Autodesk Inventor part; units mm, degrees
(part 2 of 2)
sketch "Sketch_86" plane through (0, 5.25, 0) normal (0, 1, 0) x (1, 0, 0)
  arc A0 (-220.5, -32) -> (-192.5, -60) centre (-192.5, -32) ccw
  line L0 (-192.5, -60) -> (192.5, -60)
  arc A1 (192.5, -60) -> (220.5, -32) centre (192.5, -32) ccw
  line L1 (220.5, -32) -> (220.5, 55)
  arc A2 (220.5, 55) -> (192.5, 83) centre (192.5, 55) ccw
  line L2 (192.5, 83) -> (-192.5, 83)
  arc A3 (-192.5, 83) -> (-220.5, 55) centre (-192.5, 55) ccw
  line L3 (-220.5, 55) -> (-220.5, -32)
  circle A4 centre (215.5, 11.5) radius 2.2
  circle A5 centre (174, -55) radius 2.2
  circle A6 centre (174, 78) radius 2.2
  circle A7 centre (60, -55) radius 2.2
  circle A8 centre (60, 78) radius 2.2
  circle A9 centre (-60, -55) radius 2.2
  circle A10 centre (-60, 78) radius 2.2
  circle A11 centre (-174, -55) radius 2.2
  circle A12 centre (-174, 78) radius 2.2
  arc A13 (-205.5, -37) -> (-197.5, -45) centre (-197.5, -37) ccw
  line L4 (-197.5, -45) -> (197.5, -45)
  arc A14 (197.5, -45) -> (205.5, -37) centre (197.5, -37) ccw
  line L5 (205.5, -37) -> (205.5, 60)
  arc A15 (205.5, 60) -> (197.5, 68) centre (197.5, 60) ccw
  line L6 (197.5, 68) -> (-197.5, 68)
  arc A16 (-197.5, 68) -> (-205.5, 60) centre (-197.5, 60) ccw
  line L7 (-205.5, 60) -> (-205.5, -37)
  circle A17 centre (-215.5, 11.5) radius 2.2
  constraints: 18 centre point, 16 end point, 16 point on circle
extrude "Extrusion31" add sketch "Sketch_86" against normal blind 1.25
sketch "Sketch_83" plane through (0, 0, 12.25) normal (0, 0, 1) x (1, 0, 0)
  line L0 (248.75, 17.25) -> (228.35, 17.25)
  line L1 (228.35, 17.25) -> (228.35, 20.483)
  line L2 (228.35, 20.483) -> (229.117, 21.25)
  line L3 (229.117, 21.25) -> (243.35, 21.25)
  line L4 (243.35, 21.25) -> (243.35, 23)
  line L5 (243.35, 23) -> (244.25, 23)
  line L6 (244.25, 23) -> (244.25, 24.25)
  line L7 (244.25, 24.25) -> (246.75, 24.25)
  line L8 (246.75, 24.25) -> (247.95, 22.25)
  line L9 (247.95, 22.25) -> (248.75, 22.25)
  line L10 (248.75, 22.25) -> (248.75, 17.25)
  line L11 (248.75, 17.25) -> (228.35, 17.25)
  constraints: 24 end point
revolve "Revolution35" add sketch "Sketch_83" angle 360 about axis through (248.75, 17.25, 12.25) along (-1, 0, 0)
thread "Thread5" size "M8x1.25" class "6g" standard "ISO Metric profile" length 12.983
sketch "Sketch_108" plane through (0, 0, 89.25) normal (0, 0, 1) x (1, 0, 0)
  line L0 (232.65, 437.5) -> (226.45, 437.5)
  line L1 (226.45, 437.5) -> (226.45, 442)
  line L2 (226.45, 442) -> (228.25, 442)
  line L3 (228.25, 442) -> (228.25, 440.5)
  line L4 (228.25, 440.5) -> (228.95, 440.5)
  line L5 (228.95, 440.5) -> (228.95, 440)
  line L6 (228.95, 440) -> (232.1595, 440)
  line L7 (232.1595, 440) -> (232.65, 439.5095)
  line L8 (232.65, 439.5095) -> (232.65, 437.5)
  line L9 (232.65, 437.5) -> (226.45, 437.5)
  constraints: 20 end point
revolve "Revolution36" add sketch "Sketch_108" angle 360 about axis through (232.65, 437.5, 89.25) along (1, 0, 0)
thread "Thread6" size "M5x0.8" class "6g" standard "ISO Metric profile" full length
sketch "Sketch_109" plane through (0, 0, 89.25) normal (0, 0, 1) x (1, 0, 0)
  line L0 (232.65, 62.5) -> (226.45, 62.5)
  line L1 (226.45, 62.5) -> (226.45, 67)
  line L2 (226.45, 67) -> (228.25, 67)
  line L3 (228.25, 67) -> (228.25, 65.5)
  line L4 (228.25, 65.5) -> (228.95, 65.5)
  line L5 (228.95, 65.5) -> (228.95, 65)
  line L6 (228.95, 65) -> (232.1595, 65)
  line L7 (232.1595, 65) -> (232.65, 64.5095)
  line L8 (232.65, 64.5095) -> (232.65, 62.5)
  line L9 (232.65, 62.5) -> (226.45, 62.5)
  constraints: 20 end point
revolve "Revolution37" add sketch "Sketch_109" angle 360 about axis through (232.65, 62.5, 89.25) along (1, 0, 0)
thread "Thread7" size "M5x0.8" class "6g" standard "ISO Metric profile" full length
sketch "Sketch73" plane through (247.5, 2.5, -105) normal (0, 0, -1) x (-1, 0, 0)
  point P0 (7.5, 60)
hole "Hole5" at (240, 62.5, -105) direction (0, 0, 1) diameter 10 depth 1.25
pattern_linear "Rectangular Pattern1" count 3 spacing 187.5 along (0, 1, 0) count 2 spacing 480 along (-1, 0, 0) of "Hole5"
sketch "Sketch74" plane through (247.5, 2.5, -105) normal (0, 0, -1) x (-1, 0, 0)
  point P0 (60, 7.5)
hole "Hole6" at (187.5, 10, -105) direction (0, 0, 1) diameter 10 depth 1.25
pattern_linear "Rectangular Pattern2" count 2 spacing 480 along (0, 1, 0) count 3 spacing 187.5 along (-1, 0, 0) of "Hole6"
sketch "Sketch75" plane through (-247.5, 497.5, 82) normal (0, 0, 1) x (1, 0, 0)
  point P0 (487.5, -435)
hole "Hole7" at (240, 62.5, 82) direction (0, 0, -1) diameter 10 depth 1.25
pattern_linear "Rectangular Pattern3" count 3 spacing 187.5 along (0, 1, 0) count 2 spacing 480 along (-1, 0, 0) of "Hole7"
sketch "Sketch76" plane through (-247.5, 497.5, 82) normal (0, 0, 1) x (1, 0, 0)
  point P0 (435, -487.5)
hole "Hole8" at (187.5, 10, 82) direction (0, 0, -1) diameter 10 depth 1.25
pattern_linear "Rectangular Pattern4" count 2 spacing 480 along (0, 1, 0) count 3 spacing 187.5 along (-1, 0, 0) of "Hole8"
sketch "Sketch_128" plane through (0, 10, 0) normal (0, 1, 0) x (1, 0, 0)
  line L0 (187.5, 101.95) -> (187.5, 105)
  line L1 (187.5, 103.2) -> (189.902, 103.2)
  arc A0 (189.902, 103.2) -> (190.3995, 103.65) centre (189.902, 103.7) ccw
  arc A1 (191.892, 105) -> (190.3995, 103.65) centre (191.892, 103.5) ccw
  line L2 (191.892, 105) -> (193.5, 105)
  line L3 (193.5, 105) -> (193.5, 103.75)
  line L4 (193.5, 103.75) -> (191.6685, 103.75)
  arc A2 (191.6685, 103.75) -> (190.7741, 103.1972) centre (191.6685, 102.75) ccw
  line L5 (190.7741, 103.1972) -> (190.551, 102.751)
  arc A3 (189.571, 101.95) -> (190.551, 102.751) centre (189.571, 102.95) ccw
  line L6 (189.571, 101.95) -> (187.5, 101.95)
  line L7 (187.5, 101.95) -> (187.5, 103.2)
  constraints: 16 end point, 8 point on circle, 4 centre point
revolve "Revolution38" add sketch "Sketch_128" angle 360 about axis through (187.5, 10, -101.95) along (0, 0, 1)
pattern_linear "Rectangular Pattern5" count 2 spacing 480 along (0, 1, 0) count 3 spacing 187.5 along (-1, 0, 0) of "Revolution38"
sketch "Sketch_130" plane through (0, 62.5, 0) normal (0, 1, 0) x (1, 0, 0)
  line L0 (240, 101.95) -> (240, 105)
  line L1 (240, 103.2) -> (242.402, 103.2)
  arc A0 (242.402, 103.2) -> (242.8995, 103.65) centre (242.402, 103.7) ccw
  arc A1 (244.392, 105) -> (242.8995, 103.65) centre (244.392, 103.5) ccw
  line L2 (244.392, 105) -> (246, 105)
  line L3 (246, 105) -> (246, 103.75)
  line L4 (246, 103.75) -> (244.1685, 103.75)
  arc A2 (244.1685, 103.75) -> (243.2741, 103.1972) centre (244.1685, 102.75) ccw
  line L5 (243.2741, 103.1972) -> (243.051, 102.751)
  arc A3 (242.071, 101.95) -> (243.051, 102.751) centre (242.071, 102.95) ccw
  line L6 (242.071, 101.95) -> (240, 101.95)
  line L7 (240, 101.95) -> (240, 103.2)
  constraints: 16 end point, 8 point on circle, 4 centre point
revolve "Revolution39" add sketch "Sketch_130" angle 360 about axis through (240, 62.5, -101.95) along (0, 0, 1)
pattern_linear "Rectangular Pattern6" count 3 spacing 187.5 along (0, 1, 0) count 2 spacing 480 along (-1, 0, 0) of "Revolution39"
sketch "Sketch_132" plane through (0, 10, 0) normal (0, 1, 0) x (1, 0, 0)
  line L0 (187.5, -82) -> (187.5, -78.95)
  line L1 (187.5, -78.95) -> (189.571, -78.95)
  arc A0 (190.551, -79.751) -> (189.571, -78.95) centre (189.571, -79.95) ccw
  line L2 (190.551, -79.751) -> (190.7741, -80.1972)
  arc A1 (190.7741, -80.1972) -> (191.6685, -80.75) centre (191.6685, -79.75) ccw
  line L3 (191.6685, -80.75) -> (193.5, -80.75)
  line L4 (193.5, -80.75) -> (193.5, -82)
  line L5 (193.5, -82) -> (191.892, -82)
  arc A2 (190.3995, -80.65) -> (191.892, -82) centre (191.892, -80.5) ccw
  arc A3 (190.3995, -80.65) -> (189.902, -80.2) centre (189.902, -80.7) ccw
  line L6 (189.902, -80.2) -> (187.5, -80.2)
  line L7 (187.5, -80.2) -> (187.5, -78.95)
  constraints: 16 end point, 8 point on circle, 4 centre point
revolve "Revolution40" add sketch "Sketch_132" angle 360 about axis through (187.5, 10, 82) along (0, 0, 1)
pattern_linear "Rectangular Pattern7" count 2 spacing 480 along (0, 1, 0) count 3 spacing 187.5 along (-1, 0, 0) of "Revolution40"
sketch "Sketch_134" plane through (0, 62.5, 0) normal (0, 1, 0) x (1, 0, 0)
  line L0 (240, -82) -> (240, -78.95)
  line L1 (240, -78.95) -> (242.071, -78.95)
  arc A0 (243.051, -79.751) -> (242.071, -78.95) centre (242.071, -79.95) ccw
  line L2 (243.051, -79.751) -> (243.2741, -80.1972)
  arc A1 (243.2741, -80.1972) -> (244.1685, -80.75) centre (244.1685, -79.75) ccw
  line L3 (244.1685, -80.75) -> (246, -80.75)
  line L4 (246, -80.75) -> (246, -82)
  line L5 (246, -82) -> (244.392, -82)
  arc A2 (242.8995, -80.65) -> (244.392, -82) centre (244.392, -80.5) ccw
  arc A3 (242.8995, -80.65) -> (242.402, -80.2) centre (242.402, -80.7) ccw
  line L6 (242.402, -80.2) -> (240, -80.2)
  line L7 (240, -80.2) -> (240, -78.95)
  constraints: 16 end point, 8 point on circle, 4 centre point
revolve "Revolution41" add sketch "Sketch_134" angle 360 about axis through (240, 62.5, 82) along (0, 0, 1)
pattern_linear "Rectangular Pattern8" count 3 spacing 187.5 along (0, 1, 0) count 2 spacing 480 along (-1, 0, 0) of "Revolution41"
ref_plane "FP1_XY" through (0, -0.5, -11.5) normal (0, 1, 0) x (1, 0, 0)
ref_plane "FP1_YZ" through (0, -0.5, -11.5) normal (1, 0, 0) x (0, 0, -1)
ref_plane "FP1_ZX" through (0, -0.5, -11.5) normal (0, 0, -1) x (0, 1, 0)
ref_plane "FP2_XY" through (0, -0.5, -11.5) normal (0, 1, 0) x (1, 0, 0)
ref_plane "FP2_YZ" through (0, -0.5, -11.5) normal (1, 0, 0) x (0, 0, -1)
ref_plane "FP2_ZX" through (0, -0.5, -11.5) normal (0, 0, -1) x (0, 1, 0)
ref_plane "GEHAEUSE_XY" through (0, 250, -105) normal (0, 1, 0) x (1, 0, 0)
ref_plane "GEHAEUSE_YZ" through (0, 250, -105) normal (1, 0, 0) x (0, 0, -1)
ref_plane "GEHAEUSE_ZX" through (0, 250, -105) normal (0, 0, -1) x (0, 1, 0)
ref_plane "MP_XY" through (0, 25, -85) normal (0, 0, -1) x (1, 0, 0)
ref_plane "MP_YZ" through (0, 25, -85) normal (1, 0, 0) x (0, -1, 0)
ref_plane "MP_ZX" through (0, 25, -85) normal (0, -1, 0) x (0, 0, -1)
ref_plane "REVIT_XY" through (0, 0, -105) normal (0, 0, -1) x (-1, 0, 0)
ref_plane "REVIT_YZ" through (0, 0, -105) normal (-1, 0, 0) x (0, 1, 0)
ref_plane "REVIT_ZX" through (0, 0, -105) normal (0, 1, 0) x (0, 0, -1)
ref_plane "SCLM_XY" through (-229.5, 250, 89.25) normal (1, 0, 0) x (0, 0, -1)
ref_plane "SCLM_YZ" through (-229.5, 250, 89.25) normal (0, 0, -1) x (0, 1, 0)
ref_plane "SCLM_ZX" through (-229.5, 250, 89.25) normal (0, 1, 0) x (1, 0, 0)
ref_plane "SCLO_XY" through (-229.5, 437.5, 89.25) normal (1, 0, 0) x (0, 0, -1)
ref_plane "SCLO_YZ" through (-229.5, 437.5, 89.25) normal (0, 0, -1) x (0, 1, 0)
ref_plane "SCLO_ZX" through (-229.5, 437.5, 89.25) normal (0, 1, 0) x (1, 0, 0)
ref_plane "SCLU_XY" through (-229.5, 62.5, 89.25) normal (1, 0, 0) x (0, 0, -1)
ref_plane "SCLU_YZ" through (-229.5, 62.5, 89.25) normal (0, 0, -1) x (0, 1, 0)
ref_plane "SCLU_ZX" through (-229.5, 62.5, 89.25) normal (0, 1, 0) x (1, 0, 0)
ref_plane "SCRM_XY" through (229.5, 250, 89.25) normal (-1, 0, 0) x (0, 0, -1)
ref_plane "SCRM_YZ" through (229.5, 250, 89.25) normal (0, 0, -1) x (0, -1, 0)
ref_plane "SCRM_ZX" through (229.5, 250, 89.25) normal (0, -1, 0) x (-1, 0, 0)
ref_plane "SCRO_XY" through (229.5, 437.5, 89.25) normal (-1, 0, 0) x (0, 0, -1)
ref_plane "SCRO_YZ" through (229.5, 437.5, 89.25) normal (0, 0, -1) x (0, -1, 0)
ref_plane "SCRO_ZX" through (229.5, 437.5, 89.25) normal (0, -1, 0) x (-1, 0, 0)
ref_plane "SCRU_XY" through (229.5, 62.5, 89.25) normal (-1, 0, 0) x (0, 0, -1)
ref_plane "SCRU_YZ" through (229.5, 62.5, 89.25) normal (0, 0, -1) x (0, -1, 0)
ref_plane "SCRU_ZX" through (229.5, 62.5, 89.25) normal (0, -1, 0) x (-1, 0, 0)
ref_plane "to_Abst_tzung_L_XY" through (-200, 25, -76.75) normal (0, 0, 1) x (1, 0, 0)
ref_plane "to_Abst_tzung_L_YZ" through (-200, 25, -76.75) normal (1, 0, 0) x (0, 1, 0)
ref_plane "to_Abst_tzung_L_ZX" through (-200, 25, -76.75) normal (0, 1, 0) x (0, 0, 1)
ref_plane "to_Abst_tzung_R_XY" through (200, 25, -76.75) normal (0, 0, 1) x (1, 0, 0)
ref_plane "to_Abst_tzung_R_YZ" through (200, 25, -76.75) normal (1, 0, 0) x (0, 1, 0)
ref_plane "to_Abst_tzung_R_ZX" through (200, 25, -76.75) normal (0, 1, 0) x (0, 0, 1)
ref_plane "to_Cap_1_XY" through (230, 20, -105) normal (0, 0, 1) x (1, 0, 0)
ref_plane "to_Cap_1_YZ" through (230, 20, -105) normal (1, 0, 0) x (0, 1, 0)
ref_plane "to_Cap_1_ZX" through (230, 20, -105) normal (0, 1, 0) x (0, 0, 1)
ref_plane "to_Cap_2_XY" through (-230, 20, -105) normal (0, 0, 1) x (1, 0, 0)
ref_plane "to_Cap_2_YZ" through (-230, 20, -105) normal (1, 0, 0) x (0, 1, 0)
ref_plane "to_Cap_2_ZX" through (-230, 20, -105) normal (0, 1, 0) x (0, 0, 1)
ref_plane "to_Cap_3_XY" through (230, 480, -105) normal (0, 0, 1) x (1, 0, 0)
ref_plane "to_Cap_3_YZ" through (230, 480, -105) normal (1, 0, 0) x (0, 1, 0)
ref_plane "to_Cap_3_ZX" through (230, 480, -105) normal (0, 1, 0) x (0, 0, 1)
ref_plane "to_Cap_4_XY" through (-230, 480, -105) normal (0, 0, 1) x (1, 0, 0)
ref_plane "to_Cap_4_YZ" through (-230, 480, -105) normal (1, 0, 0) x (0, 1, 0)
ref_plane "to_Cap_4_ZX" through (-230, 480, -105) normal (0, 1, 0) x (0, 0, 1)
ref_plane "to_Plug_XY" through (-233.5, 0, 65.5) normal (0, 1, 0) x (1, 0, 0)
ref_plane "to_Plug_YZ" through (-233.5, 0, 65.5) normal (1, 0, 0) x (0, 0, -1)
ref_plane "to_Plug_ZX" through (-233.5, 0, 65.5) normal (0, 0, -1) x (0, 1, 0)
ref_plane "to_Plug_3_XY" through (200, 500, 16.5) normal (0, 1, 0) x (1, 0, 0)
ref_plane "to_Plug_3_YZ" through (200, 500, 16.5) normal (1, 0, 0) x (0, 0, -1)
ref_plane "to_Plug_3_ZX" through (200, 500, 16.5) normal (0, 0, -1) x (0, 1, 0)
ref_plane "to_Plug_4_XY" through (-200, 500, 16.5) normal (0, 1, 0) x (1, 0, 0)
ref_plane "to_Plug_4_YZ" through (-200, 500, 16.5) normal (1, 0, 0) x (0, 0, -1)
ref_plane "to_Plug_4_ZX" through (-200, 500, 16.5) normal (0, 0, -1) x (0, 1, 0)
ref_plane "to_Plug_1_1_XY" through (205, 0, -60) normal (0, 1, 0) x (1, 0, 0)
ref_plane "to_Plug_1_1_YZ" through (205, 0, -60) normal (1, 0, 0) x (0, 0, -1)
ref_plane "to_Plug_1_1_ZX" through (205, 0, -60) normal (0, 0, -1) x (0, 1, 0)
ref_plane "to_Plug_1_2_XY" through (-205, 0, -60) normal (0, 1, 0) x (1, 0, 0)
ref_plane "to_Plug_1_2_YZ" through (-205, 0, -60) normal (1, 0, 0) x (0, 0, -1)
ref_plane "to_Plug_1_2_ZX" through (-205, 0, -60) normal (0, 0, -1) x (0, 1, 0)
ref_plane "to_Plug_1_3_XY" through (205, 0, 127.5) normal (0, 1, 0) x (1, 0, 0)
ref_plane "to_Plug_1_3_YZ" through (205, 0, 127.5) normal (1, 0, 0) x (0, 0, -1)
ref_plane "to_Plug_1_3_ZX" through (205, 0, 127.5) normal (0, 0, -1) x (0, 1, 0)
ref_plane "to_Plug_1_4_XY" through (-205, 0, 127.5) normal (0, 1, 0) x (1, 0, 0)
ref_plane "to_Plug_1_4_YZ" through (-205, 0, 127.5) normal (1, 0, 0) x (0, 0, -1)
ref_plane "to_Plug_1_4_ZX" through (-205, 0, 127.5) normal (0, 0, -1) x (0, 1, 0)
body "Solid1"
